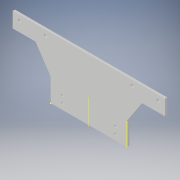
# Autodesk Inventor part: plate
Saved by Autodesk Inventor 2017 (Build 210142000, 142)
## iProperties
Created: 2017-04-05
Part Number: plate
Material: Generic
Document SubType Name: Modeling
Designer: s4461999
Density: 1 g/cm^3
Appearance: Default
Author: s4461999
Autodesk Inventor part; units mm, degrees
ref_plane "YZ Plane" through (0, 0, 0) normal (1, 0, 0) x (0, 1, 0)
ref_plane "XZ Plane" through (0, 0, 0) normal (0, 1, 0) x (-1, 0, 0)
ref_plane "XY Plane" through (0, 0, 0) normal (0, 0, 1) x (1, 0, 0)
sketch "Sketch1" plane through (0, 0, 0) normal (0, 1, 0) x (-1, 0, 0)
  point P0 (0, 0)
sketch "Sketch2" plane through (0, 0, 0) normal (0, 0, 1) x (1, 0, 0)
  line L0 (0, 0) -> (100, 0)
  line L1 (100, 0) -> (100, 30)
  line L2 (100, 30) -> (120, 60)
  line L3 (120, 60) -> (150, 60)
  line L4 (150, 60) -> (150, 80)
  line L5 (150, 80) -> (-50, 80)
  line L6 (-50, 80) -> (-50, 60)
  line L7 (0, 30) -> (0, 0)
  line L8 (-50, 60) -> (-20, 60)
  line L9 (-20, 60) -> (0, 30)
  dimension "d0" = 100
  dimension "d1" = 200
  dimension "d2" = 0
  dimension "d3" = 20
  dimension "d4" = 30
  dimension "d5" = 30
  dimension "d6" = 20
  dimension "d7" = 30
  dimension "d8" = 30
  dimension "d9" = 20
  dimension "d10" = 20
  constraints: 20 end point, 3 equal length, 2 perpendicular, 1 collinear, 1 horizontal
  measures "d0" distance of L0.start L0.end
  measures "d1" distance of L4.end L5.end
  measures "d2" angle of L0 L5
  measures "d3" distance of L3.end L4.end
  measures "d4" distance of L0.end L1.end
  measures "d5" distance of L7.start L0.start
  measures "d6" distance of L5.end L6.end
  measures "d7" distance from line of L3 L1.end
  measures "d8" vertical distance of L7.start L8.end
  measures "d9" horizontal distance of L8.end L7.start
  measures "d10" horizontal distance of L2.end L1.end
sketch "Sketch3" plane through (0, 0, 0) normal (0, 0, 1) x (1, 0, 0)
  point P0 (0, 0)
sketch "Sketch4" plane through (0, 0, 0) normal (0, 0, 1) x (1, 0, 0)
  point P0 (0, 0)
extrude "Extrusion1" add sketch "Sketch2" along normal blind 3
sketch "Sketch6" plane through (0, 0, 3) normal (0, 0, 1) x (1, 0, 0)
  point P0 (0, 0)
sketch "Sketch7" plane through (0, 0, 0) normal (0, 0, -1) x (-1, 0, 0)
  point P0 (0, 0)
sketch "Sketch8" plane through (0, 0, 3) normal (0, 0, 1) x (1, 0, 0)
  point P0 (0, 0)
sketch "Sketch9" plane through (0, 0, 3) normal (0, 0, 1) x (1, 0, 0)
  line L0 (-50, 80) -> (-50, 60) projected
  line L1 (150, 80) -> (-50, 80) projected
  line L2 (0, 30) -> (0, 0) projected
  line L3 (0, 0) -> (100, 0) projected
  point P0 (15, 16)
  point P1 (15, 7)
  dimension "d37" = 15
  dimension "d38" = 15
  dimension "d39" = 7
  dimension "d40" = 9
  measures "d37" distance from line of point (15, 16) L2
  measures "d38" distance from line of point (15, 7) L2
  measures "d39" distance from line of point (15, 7) L3
  measures "d40" distance of point (15, 7) point (15, 16)
hole "Hole2" at (15, 7, 3) at (15, 16, 3) direction (0, 0, -1) diameter 3.4 end through all
sketch "Sketch11" plane through (0, 0, 3) normal (0, 0, 1) x (1, 0, 0)
  line L0 (100, 0) -> (100, 30) projected
  point P0 (0, 0)
sketch "Sketch12" plane through (0, 0, 3) normal (0, 0, 1) x (1, 0, 0)
  line L0 (-50, 80) -> (-50, 60) projected
  line L1 (150, 80) -> (-50, 80) projected
  point P0 (0, 0)
  point P1 (-41, 73)
  point P2 (-7, 73)
  dimension "d50" = 9
  dimension "d51" = 34
  dimension "d52" = 7
  dimension "d53" = 7
  measures "d50" distance from line of point (-41, 73) L0
  measures "d51" distance of point (-7, 73) point (-41, 73)
  measures "d52" distance from line of point (-41, 73) L1
  measures "d53" distance from line of point (-7, 73) L1
hole "Hole3" at (-41, 73, 3) at (-7, 73, 3) direction (0, 0, -1) diameter 4.4 end through all
ref_plane "Work Plane2" through (50, 0, 0) normal (-1, 0, 0) x (0, 0, 1)
mirror "Mirror1" about plane through (50, 0, 0) normal (-1, 0, 0) of "Hole2", "Hole3"
sketch "Sketch14" plane through (0, 0, 3) normal (0, 0, 1) x (1, 0, 0)
  point P0 (0, 0)
sketch "Sketch15" plane through (0, 0, 3) normal (0, 0, 1) x (1, 0, 0)
  point P0 (0, 0)
sketch "Sketch16" plane through (0, 0, 3) normal (0, 0, 1) x (1, 0, 0)
  point P0 (0, 0)
body "Solid1"
